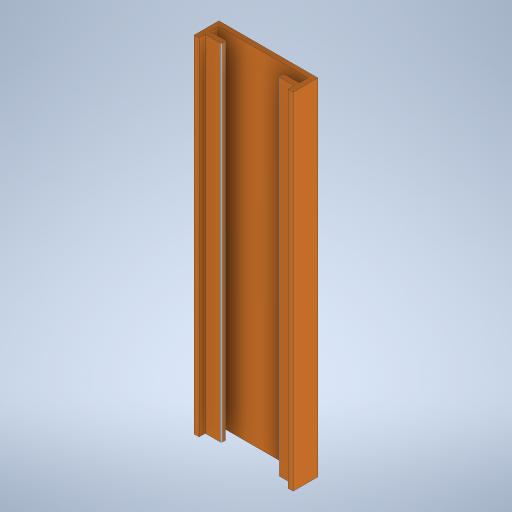
# Autodesk Inventor part: lift
Saved by Autodesk Inventor 2024 (Build 280153000, 153)
## iProperties
Created: 2024-03-13
Part Number: lift
Material: Generic
Document SubType Name: Modeling
Designer: dustp
Density: 1 g/cm^3
Appearance: Default
Author: dustp
Autodesk Inventor part; units mm, degrees
ref_plane "YZ Plane" through (0, 0, 0) normal (1, 0, 0) x (0, 1, 0)
ref_plane "XZ Plane" through (0, 0, 0) normal (0, 1, 0) x (-1, 0, 0)
ref_plane "XY Plane" through (0, 0, 0) normal (0, 0, 1) x (1, 0, 0)
sketch "Sketch1" plane through (0, 0, 0) normal (0, 1, 0) x (-1, 0, 0)
  line L0 (0, 0) -> (-40, 0)
  line L1 (-40, 0) -> (-40, -10)
  line L2 (-40, -10) -> (0, -10)
  line L3 (0, -10) -> (0, 0)
  line L4 (0, 0) -> (-40, 0)
  line L5 (-40, 0) -> (-40, -2)
  line L6 (-40, -2) -> (0, -2)
  line L7 (0, -2) -> (0, 0)
  line L8 (0, -10) -> (-2, -10)
  line L9 (-2, -10) -> (-2, 0)
  line L10 (-2, 0) -> (0, 0)
  line L11 (0, 0) -> (0, -10)
  line L12 (-40, -10) -> (-38, -10)
  line L13 (-38, -10) -> (-38, 0)
  line L14 (-38, 0) -> (-40, 0)
  line L15 (-40, 0) -> (-40, -10)
  line L16 (-2, -7.5) -> (-38, -7.5)
  line L17 (-38, -7.5) -> (-38, -5.5)
  line L18 (-38, -5.5) -> (-2, -5.5)
  line L19 (-2, -5.5) -> (-2, -7.5)
  line L20 (-8.5, -10) -> (-31.5, -10)
  line L21 (-31.5, -10) -> (-31.5, -2)
  line L22 (-31.5, -2) -> (-8.5, -2)
  line L23 (-8.5, -2) -> (-8.5, -10)
  point P0 (-38, -10)
  point P1 (-38, -7.5)
  point P2 (-31.5, -7.5)
  point P3 (-31.5, -5.5)
  point P4 (-38, -2)
  point P5 (-2, -2)
  point P6 (-2, -5.5)
  point P7 (-8.5, -5.5)
  point P8 (-8.5, -7.5)
  dimension "d0" = 10
  dimension "d1" = 40
  dimension "d2" = 2
  dimension "d3" = 2
  dimension "d4" = 2
  dimension "d5" = 2
  dimension "d6" = 3.5
  dimension "d7" = 2.5
  dimension "d13" = 6.5
  dimension "d14" = 6.5
  constraints: 48 end point, 12 parallel, 7 point on line, 6 horizontal, 6 perpendicular
  measures "d0" distance of L2.end L0.start
  measures "d1" distance of L1.end L2.end
  measures "d2" distance of L5.end L4.end
  measures "d3" distance of L9.end L10.end
  measures "d4" distance of L14.end L13.end
  measures "d5" distance of L16.end L17.end
  measures "d6" distance between parallel lines of L6 L18
  measures "d7" distance between parallel lines of L2 L16
  measures "d13" distance between parallel lines of L9 L23
  measures "d14" distance between parallel lines of L21 L13
extrude "Extrusion1" add sketch "Sketch1" along normal blind 139.7 contours L3 L6 L9 L0 | L9 L6 L13 L0 | L3 L2 L9 L6 | L13 L6 L1 L0 | L13 L2 L1 L6 | L9 L16 L23 L18 | L18 L21 L16 L13
fillet "Fillet1" radius 0.5 2 edges at (31.5, 69.85, -7.5) (31.5, 69.85, -5.5)
fillet "Fillet2" radius 0.5 2 edges at (8.5, 69.85, -5.5) (8.5, 69.85, -7.5)
move or copy body "Rotate1" bodies to move or copy 1 copy no rotation origin (0, 0, 0) rotation axis (0, 1, 0) rotation angle 180 translate (40, 0, 0)
body "Solid1"
